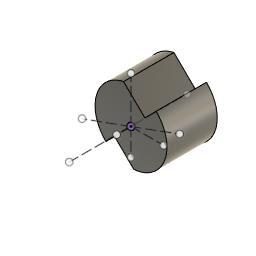
AAA-Revolver (Autodesk Fusion 360 design; units mm, degrees)
Autodesk Fusion 360 part; units mm, degrees
sketch "Skizze4" plane through (0, 0, 0) normal (1, 0, 0) x (0, 1, 0)
  line L0 (-43, 0) -> (39, 0) construction
  line L1 (0, 0) -> (-10, 0) construction
  line L2 (0, 0) -> (0, 32) construction
  line L3 (0, 0) -> (0, -18.5834) construction
  constraint horizontal L0
  constraint coincident L1.start L2.start
  constraint horizontal L1
  constraint collinear L0 L1
  constraint collinear L2 L3
  constraint vertical L2
sketch "Skizze5" plane through (0, 0, 0) normal (0, 1, 0) x (1, 0, 0)
  line L0 (0, 0) -> (-34.0577, 12.396) construction
  line L1 (0, 0) -> (33.8638, -12.3254) construction
  line L2 (0, 0) -> (22.8035, 0) construction
  dimension "d18" = 20
  constraint coincident L0.start L1.start
  constraint horizontal L2
  constraint collinear L0 L1
  measures "d18" angle of L1 L2
sketch "Skizze1" plane through (0, 0, 0) normal (0, 1, 0) x (1, 0, 0)
  circle A0 centre (0, 0) radius 25
  circle A1 centre (0, 0) radius 2.25
  dimension "d1" = 50
  dimension "d14" = 4.5
  constraint coincident A0.centre A1.centre
  measures "d1" diameter of A0
  measures "d14" diameter of A1
extrude "Extrusion1" add sketch "Skizze1" along normal mid plane 35 makes body 1
sketch "Skizze2" plane through (0, -17.5, 0) normal (0, -1, 0) x (1, 0, 0)
  circle A0 centre (0, 0) radius 25
  line L0 (0, 0) -> (85.163, 30.9968) construction
  line L1 (0, 0) -> (100, 0) construction
  circle A1 centre (17.2047, 13.7112) radius 7
  line L2 (17.2047, 13.7112) -> (82.8425, 37.6015) construction
  circle A2 centre (0, 0) radius 29 construction
  line L3 (0, 0) -> (-43.7134, -15.9104) construction
  line L4 (13.021, 4.7393) -> (5.9041, 24.2928)
  line L5 (13.021, 4.7393) -> (23.4923, 8.5505)
  circle A3 centre (0, 0) radius 2.25
  circle A4 centre (17.2047, 13.7112) radius 1
  circle A5 centre (0, 0) radius 27 construction
  line L6 (-42.6624, -20.8487) -> (-6.6953, -7.7578) construction
  circle A6 centre (-18.4221, -12.026) radius 5
  line L7 (-18.4221, -12.026) -> (-54.0112, -24.9794) construction
  line L8 (-15.4338, -5.6174) -> (-8.9874, -23.3287)
  line L9 (-23.4923, -8.5505) -> (-15.4338, -5.6174)
  circle A7 centre (-18.4221, -12.026) radius 1
  dimension "d5" = 20
  dimension "d6" = 14
  dimension "d7" = 7
  dimension "d10" = 50
  dimension "d11" = 58
  dimension "d41" = 2
  dimension "d42" = 54
  dimension "d43" = 5
  dimension "d44" = 10
  dimension "d45" = 2
  constraint horizontal L1
  constraint coincident A0.centre L0.start
  constraint coincident A1.centre L2.start
  constraint tangent A1 A2
  constraint collinear L0 L3
  constraint coincident L0 L4.start
  constraint coincident A0 L4.end
  constraint perpendicular L0 L4
  constraint tangent A1 L4
  constraint coincident L0 L5.end
  constraint coincident A0 L5.end
  constraint concentric A1 A4
  constraint parallel L3 L6
  constraint coincident A6.centre L7.start
  constraint collinear L6 L7
  constraint tangent A5 A6
  constraint coincident L3 L8.start
  constraint coincident A0 L8.end
  constraint perpendicular L6 L8
  constraint tangent A6 L8
  constraint coincident L3 L9.start
  constraint coincident A0 L9.start
  constraint concentric A6 A7
  measures "d5" angle of L0 L1
  measures "d6" diameter of A1
  measures "d7" distance of L0 L2
  measures "d10" diameter of A0
  measures "d11" diameter of A2
  measures "d41" diameter of A4
  measures "d42" diameter of A5
  measures "d43" distance of L3 L6
  measures "d44" diameter of A6
  measures "d45" diameter of A7
extrude "Extrusion6" cut sketch "Skizze2" against normal blind 35 contours A0 A1 L5 | A0 A6 L8 | A0 A1 | A1 L4 L5 | A0 A6 | A6 L8 L9 | A0 A1 L4 | A0 A6 L9 | A4 | A7 picked at (20.1527, 11.2218) picked at (-18.6926, -14.9391) bodies 1
extrude "Extrusion7" add sketch "Skizze2" against normal blind 35 separate body contours A0 A1 | A0 A1 | A0 A6 | A0 A6 makes body 2 at (24.196, 5.8333, 13.3623) makes body 3 at (-13.4284, 5.8333, -12.2752)
copy_body "Körper->Berechn9" bodies 1 removing the originals makes body 4 in component "Revolver"
copy_body "Körper->Berechn10" bodies 2 removing the originals makes body 5 in component "AA"
copy_body "Körper->Berechn11" bodies 3 removing the originals makes body 6 in component "AAA"
component "Revolver" placed x (1, 0, 0) y (0, 1, 0) z (0, 0, 1) at (0, 17.5, 0)
component "AA" placed x (1, 0, 0) y (0, 1, 0) z (0, 0, 1) at (0, 0, 0)
component "AAA" placed x (1, 0, 0) y (0, 1, 0) z (0, 0, 1) at (0, 0, 0)
hidden bodies 5 6
equation "d11 = d10 + 8 mm"
equation "d42 = d10 + 4 mm"
named bodies: "Revolver", "AA", "AAA"
